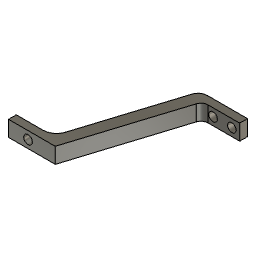
ヘイロー_ジョイント_mk1 v2 (Autodesk Fusion 360 archive; units mm, degrees)
design "ヘイロー　ジョイント　アクリル"
Autodesk Fusion 360 part; units mm, degrees
sketch "スケッチ1" plane through (0, 0, 0) normal (0, 0, 1) x (1, 0, 0)
  line L0 (25, 10) -> (44.6738, 72.577)
  line L1 (0, 0) -> (29.8739, 0)
  line L2 (75.9944, 76.7775) -> (71.9944, 76.7775)
  line L3 (50.3976, 76.7775) -> (57.9944, 76.7775)
  line L4 (75.9944, 76.7775) -> (75.9944, 71.7775)
  line L5 (75.9944, 71.7775) -> (55.7427, 71.7775)
  line L6 (51.4498, 68.6271) -> (29.8739, 0)
  line L7 (0, 0) -> (0, 5)
  line L8 (0, 5) -> (11.5, 5)
  line L9 (13.5, 5) -> (17.1902, 5)
  line L10 (25, 10) -> (25.2989, 10.9507)
  arc A0 (55.7427, 71.7775) -> (51.4498, 68.6271) centre (55.7427, 67.2775) ccw
  arc A1 (50.3976, 76.7775) -> (44.6738, 72.577) centre (50.3976, 70.7775) ccw
  arc A2 (17.1902, 5) -> (25.2989, 10.9507) centre (17.1902, 13.5) ccw
  line L11 (11.5, 5) -> (13.5, 5)
  line L12 (57.9944, 76.7775) -> (71.9944, 76.7775)
  point P0 (45.9944, 76.7775)
  dimension "d3" = 70
  dimension "d4" = 30
  dimension "d7" = 4
  dimension "d18" = 5
  dimension "d19" = 11.5
  dimension "d22" = 4.5
  dimension "d23" = 6
  dimension "d24" = 8.5
  constraint coincident L1.start L7.start
  constraint perpendicular L2 L4
  constraint perpendicular L4 L5
  constraint perpendicular L1 L7
  constraint perpendicular L7 L8
  constraint parallel L0 L10
  constraint tangent L6 A0
  constraint tangent L5 A0
  constraint coincident P0 L0
  constraint coincident P0 L3
  constraint tangent L0 A1
  constraint tangent L3 A1
  constraint tangent L10 A2
  constraint tangent L9 A2
  constraint parallel L9 L11
  constraint parallel L2 L12
  measures "d3" distance of L0.start P0
  measures "d4" distance of P0 L2.start
  measures "d7" distance of L2.start L2.end
  measures "d18" distance of L2.start L4.end
  measures "d19" distance of L7.end L8.end
  measures "d22" radius of A0
  measures "d23" radius of A1
  measures "d24" radius of A2
extrude "押し出し1" add sketch "スケッチ1" along normal blind 10 makes body 1
sketch "スケッチ2" plane through (0, 76.7775, 0) normal (0, 1, 0) x (-1, 0, 0)
  line L0 (-69.9944, 0) -> (-59.9944, 0)
  line L1 (-59.9944, 0) -> (-59.9944, 10)
  line L2 (-59.9944, 10) -> (-69.9944, 10)
  line L3 (-69.9944, 10) -> (-69.9944, 0)
  circle A0 centre (-71, 5) radius 2.75
  circle A1 centre (-59, 5) radius 2.75
  circle A2 centre (-12.5, 5) radius 2.75
  dimension "d31" = 5.5
  dimension "d32" = 5.5
  dimension "d33" = 5.5
  measures "d31" diameter of A0
  measures "d32" diameter of A1
  measures "d33" diameter of A2
extrude "押し出し2" add sketch "スケッチ1" along normal blind 10 separate body makes body 2
extrude "押し出し3" cut sketch "スケッチ2" against normal blind 105 contours L3 A0 | L3 A0 | L1 A1 | L1 A1 | A2 bodies 1 2
combine "結合1" operation add target body 1 tool bodies 2
